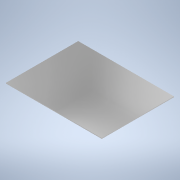
# Autodesk Inventor part: Pieza26
Saved by Autodesk Inventor 2022.2 (Build 262287000, 287)
## iProperties
Created: 2022-02-11
Part Number: Pieza26
Material: Aluminio 6061
Document SubType Name: Modeling
Designer: USUARIO
Mass: 4298.22 g
Surface Area: 6485.51 cm^2
Volume: 1591.93 cm^3
Density: 2.7 g/cm^3
Appearance: Aluminio - Plano
Author: USUARIO
Autodesk Inventor part; units mm, degrees
ref_plane "YZ Plane" through (0, 0, 0) normal (1, 0, 0) x (0, 1, 0)
ref_plane "XZ Plane" through (0, 0, 0) normal (0, 1, 0) x (-1, 0, 0)
ref_plane "XY Plane" through (0, 0, 0) normal (0, 0, 1) x (1, 0, 0)
sketch "Boceto1" plane through (0, 0, 0) normal (0, 1, 0) x (-1, 0, 0)
  line L0 (662.5132, 1844.5674) -> (12.5132, 1844.5674)
  line L1 (12.5132, 1844.5674) -> (12.5132, 1354.5674)
  line L2 (12.5132, 1354.5674) -> (662.5132, 1354.5674)
  line L3 (662.5132, 1354.5674) -> (662.5132, 1844.5674)
  point P0 (0, 0)
  dimension "d0" = 650
  dimension "d1" = 490
  constraints: 8 end point, 2 parallel, 1 horizontal, 1 perpendicular
  measures "d0" distance of L2.end L1.end
  measures "d1" distance of L1.end L0.end
extrude "Extrusión1" add sketch "Boceto1" along normal blind 5
sketch "Boceto2" plane through (0, 5, 0) normal (0, 1, 0) x (1, 0, 0)
  arc A0 (-288.7292, -1279.5674) -> (-301.2292, -1279.5674) centre (-294.9792, -1279.5674) ccw projected
  circle A1 centre (-548.8292, -1364.5674) radius 3
  circle A2 centre (-476.1292, -1364.5674) radius 3
  circle A3 centre (-476.1292, -1454.5674) radius 3
  circle A4 centre (-548.8292, -1454.5674) radius 3
  point P0 (0, 0)
  dimension "d6" = 6
  dimension "d7" = 253.85
  dimension "d9" = 6
  dimension "d10" = 72.7
  dimension "d11" = 6
  dimension "d12" = 6
  dimension "d13" = 90
  dimension "d14" = 90
  constraints: 4 centre point, 2 vertical alignment
  measures "d6" diameter of A1
  measures "d7" horizontal distance of A0.centre A1.centre
  measures "d9" diameter of A2
  measures "d10" distance of A1.centre A2.centre
  measures "d11" diameter of A3
  measures "d12" diameter of A4
  measures "d13" distance of A1.centre A4.centre
  measures "d14" distance of A2.centre A3.centre
extrude "Extrusión3" cut sketch "Boceto2" against normal through all
sketch "Boceto3" plane through (0, 5, 0) normal (0, 1, 0) x (1, 0, 0)
  line L0 (-502.9542, -1515.5674) -> (-522.0042, -1515.5674) projected
  line L1 (-607.4792, -1534.5674) -> (-417.4792, -1534.5674)
  line L2 (-417.4792, -1534.5674) -> (-417.4792, -1774.5674)
  line L3 (-417.4792, -1774.5674) -> (-607.4792, -1774.5674)
  line L4 (-607.4792, -1774.5674) -> (-607.4792, -1534.5674)
  line L5 (-662.5132, -1844.5674) -> (-12.5132, -1844.5674) projected
  point P0 (0, 0)
  point P1 (-512.4792, -1534.5674)
  point P2 (-512.4792, -1515.5674)
  dimension "d17" = 190
  dimension "d18" = 240
  dimension "d19" = 70
  constraints: 8 end point, 2 midpoint, 2 parallel, 1 horizontal, 1 perpendicular, 1 vertical alignment
  measures "d17" distance of L2.end L3.end
  measures "d18" distance of L1.end L2.end
  measures "d19" distance between parallel lines of L3 L5
extrude "Extrusión4" cut sketch "Boceto3" against normal through all
